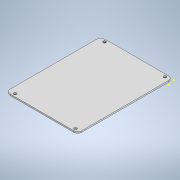
# Autodesk Inventor part: Base
Saved by Autodesk Inventor 2022 (Build 260153000, 153)
## iProperties
Created: 2021-07-02
Part Number: Base
Material: Generic
Document SubType Name: Modeling
Designer: anton
Density: 1 g/cm^3
Appearance: Default
Author: anton
Autodesk Inventor part; units mm, degrees
ref_plane "YZ Plane" through (0, 0, 0) normal (1, 0, 0) x (0, 1, 0)
ref_plane "XZ Plane" through (0, 0, 0) normal (0, 1, 0) x (-1, 0, 0)
ref_plane "XY Plane" through (0, 0, 0) normal (0, 0, 1) x (1, 0, 0)
sketch "Sketch9" plane through (0, 0, 0) normal (0, 1, 0) x (-1, 0, 0)
  line L0 (21.5945, 0.4535) -> (21.5945, 2.4535)
  line L1 (17.5945, 2.4535) -> (21.5945, 2.4535)
  line L2 (17.5945, 2.4535) -> (17.5945, 10.4535)
  line L3 (17.5945, 10.4535) -> (4.5945, 10.4535)
  line L4 (4.5945, 183.6535) -> (4.5945, 10.4535)
  line L5 (4.5945, 183.6535) -> (17.5945, 183.6535)
  line L6 (17.5945, 183.6535) -> (17.5945, 191.6535)
  line L7 (128.8958, 191.6535) -> (17.5945, 191.6535)
  line L8 (128.8958, 191.6535) -> (128.8958, 183.6535)
  line L9 (128.8958, 183.6535) -> (145.8958, 183.6535)
  line L10 (145.8958, 183.6535) -> (145.8958, 77.6035)
  line L11 (145.8958, 77.6035) -> (148.4777, 77.6035)
  line L12 (148.4777, 77.6035) -> (148.4777, 185.6535)
  ellipse E0 centre (138.5419, 185.6535) end of major axis (148.4777, 185.6535) minor radius 8 (148.4777, 185.6535) -> (138.5419, 193.6535) ccw
  line L13 (138.5419, 193.6535) -> (11.132, 193.6535)
  ellipse E1 centre (11.132, 185.6535) end of major axis (2.4153, 185.6535) minor radius 8 (11.132, 193.6535) -> (2.4153, 185.6535) ccw
  line L14 (2.4153, 8.4535) -> (2.4153, 185.6535)
  ellipse E2 centre (11.132, 8.4535) end of major axis (2.4153, 8.4535) minor radius 8 (2.4153, 8.4535) -> (11.132, 0.4535) ccw
  line L15 (11.132, 0.4535) -> (21.5945, 0.4535)
  circle A0 centre (135.4777, 188.1535) radius 2.9
  circle A1 centre (12.4153, 5.9535) radius 2.9
  circle A2 centre (12.4153, 188.1535) radius 2.9
  line L16 (46.5945, 2.4535) -> (46.5945, 0.4535)
  line L17 (46.5945, 0.4535) -> (138.5419, 0.4535)
  ellipse E3 centre (138.5419, 8.4535) end of major axis (128.606, 8.4535) minor radius 8 (138.5419, 0.4535) -> (148.4777, 8.4535) ccw
  line L18 (148.4777, 8.4535) -> (148.4777, 10.4535)
  line L19 (148.4777, 10.4535) -> (128.8958, 10.4535)
  line L20 (128.8958, 10.4535) -> (128.8958, 2.4535)
  line L21 (46.5945, 2.4535) -> (128.8958, 2.4535)
  circle A3 centre (135.4777, 5.9535) radius 2.9
  point P0 (0, 0)
  point P1 (98.6744, 193.6535)
  constraints: 44 end point, 4 centre point, 16 other
extrude "Extrusion8" add sketch "Sketch9" along normal blind 3
sketch "Sketch12" plane through (0, 3, 0) normal (0, 1, 0) x (1, 0, 0)
  line L0 (-17.5945, -183.6535) -> (-17.5945, -191.6535) projected
  line L1 (-17.5945, -191.6535) -> (-128.8958, -191.6535) projected
  line L2 (-128.8958, -191.6535) -> (-128.8958, -183.6535) projected
  line L3 (-128.8958, -183.6535) -> (-145.8958, -183.6535) projected
  line L4 (-145.8958, -183.6535) -> (-145.8958, -77.6035) projected
  line L5 (-145.8958, -77.6035) -> (-148.4777, -77.6035) projected
  line L6 (-148.4777, -77.6035) -> (-148.4777, -185.6535) projected
  ellipse E0 centre (-138.5419, -185.6535) end of major axis (-148.4777, -185.6535) minor radius 8 (-148.4777, -185.6535) -> (-138.5419, -193.6535) ccw projected
  line L7 (-138.5419, -193.6535) -> (-11.132, -193.6535) projected
  ellipse E1 centre (-11.132, -185.6535) end of major axis (-2.4153, -185.6535) minor radius 8 (-11.132, -193.6535) -> (-2.4153, -185.6535) ccw projected
  line L8 (-2.4153, -185.6535) -> (-2.4153, -8.4535) projected
  ellipse E2 centre (-11.132, -8.4535) end of major axis (-2.4153, -8.4535) minor radius 8 (-2.4153, -8.4535) -> (-11.132, -0.4535) ccw projected
  line L9 (-11.132, -0.4535) -> (-21.5945, -0.4535) projected
  line L10 (-21.5945, -0.4535) -> (-21.5945, -2.4535) projected
  line L11 (-21.5945, -2.4535) -> (-17.5945, -2.4535) projected
  line L12 (-17.5945, -2.4535) -> (-17.5945, -10.4535) projected
  line L13 (-17.5945, -10.4535) -> (-4.5945, -10.4535) projected
  line L14 (-4.5945, -10.4535) -> (-4.5945, -183.6535) projected
  line L15 (-4.5945, -183.6535) -> (-17.5945, -183.6535) projected
  circle A0 centre (-135.4777, -188.1535) radius 2.9 projected
  circle A1 centre (-12.4153, -5.9535) radius 2.9 projected
  circle A2 centre (-12.4153, -188.1535) radius 2.9 projected
  line L16 (-46.5945, -0.4535) -> (-138.5419, -0.4535) projected
  ellipse E3 centre (-138.5419, -8.4535) end of major axis (-128.606, -8.4535) minor radius 8 (-138.5419, -0.4535) -> (-148.4777, -8.4535) ccw projected
  line L17 (-148.4777, -8.4535) -> (-148.4777, -10.4535) projected
  line L18 (-148.4777, -10.4535) -> (-128.8958, -10.4535) projected
  line L19 (-128.8958, -10.4535) -> (-128.8958, -2.4535) projected
  line L20 (-128.8958, -2.4535) -> (-46.5945, -2.4535) projected
  line L21 (-46.5945, -2.4535) -> (-46.5945, -0.4535) projected
  circle A3 centre (-135.4777, -5.9535) radius 2.9 projected
  line L22 (-148.4777, -77.6035) -> (-148.4777, -185.6535) projected
  line L23 (-148.4777, -77.6035) -> (-148.4777, -10.4535)
  line L24 (-46.5945, -0.4535) -> (-138.5419, -0.4535) projected
  line L25 (-11.132, -0.4535) -> (-21.5945, -0.4535) projected
  line L26 (-46.5945, -0.4535) -> (-21.5945, -0.4535)
  point P0 (0, 0)
  constraints: 4 end point, 2 collinear, 4 other
extrude "Extrusion9" add sketch "Sketch12" along normal blind 3
sketch "Sketch14" plane through (0, 3, 0) normal (0, -1, 0) x (1, 0, 0)
  line L0 (-148.4777, 8.4535) -> (-148.4777, 10.4535) projected
  line L1 (-148.4777, 10.4535) -> (-76.8917, 10.4535)
  line L2 (-76.8917, 10.4535) -> (-76.8917, 77.6035)
  line L3 (-76.8917, 77.6035) -> (-148.4777, 77.6035)
  line L4 (-148.4777, 77.6035) -> (-148.4777, 10.4535)
  circle A0 centre (-136.5827, 69.7935) radius 4
  circle A1 centre (-139.8757, 18.2635) radius 4
  circle A2 centre (-85.5757, 18.2635) radius 4
  circle A3 centre (-86.4447, 69.1635) radius 4
  point P0 (0, 0)
  dimension "d72" = 71.586
  dimension "d73" = 67.15
  dimension "d74" = 8
  dimension "d75" = 8
  dimension "d76" = 8
  dimension "d77" = 8
  dimension "d78" = 7.81
  dimension "d79" = 11.895
  dimension "d80" = 8.44
  dimension "d81" = 9.553
  dimension "d82" = 7.81
  dimension "d83" = 8.684
  dimension "d84" = 7.81
  dimension "d85" = 8.602
  constraints: 8 end point, 4 centre point, 2 parallel, 1 horizontal, 1 perpendicular
  measures "d72" distance between parallel lines of L4 L2
  measures "d73" distance between parallel lines of L1 L3
  measures "d74" diameter of A3
  measures "d75" diameter of A2
  measures "d76" diameter of A1
  measures "d77" diameter of A0
  measures "d78" distance from line of A0.centre L3
  measures "d79" distance from line of L4 A0.centre
  measures "d80" distance from line of L3 A3.centre
  measures "d81" distance from line of L2 A3.centre
  measures "d82" distance from line of L1 A2.centre
  measures "d83" distance from line of L2 A2.centre
  measures "d84" distance from line of L1 A1.centre
  measures "d85" distance from line of L4 A1.centre
extrude "Extrusion10" add sketch "Sketch14" along normal blind 3 contours A0 | A1 | A2 | A3
sketch "Sketch15" plane through (0, 3, 0) normal (0, -1, 0) x (1, 0, 0)
  line L0 (-148.4777, 10.4535) -> (-128.8958, 10.4535) projected
  line L1 (-145.8958, 77.6035) -> (-148.4777, 77.6035) projected
  line L2 (-145.9777, 10.4535) -> (-148.4777, 10.4535)
  line L3 (-148.4777, 10.4535) -> (-148.4777, 77.6035)
  line L4 (-148.4777, 77.6035) -> (-145.9777, 77.6035)
  line L5 (-145.9777, 77.6035) -> (-145.9777, 10.4535)
  point P0 (0, 0)
  dimension "d88" = 2.5
  constraints: 8 end point, 2 parallel, 1 horizontal, 1 perpendicular, 1 point on line
  measures "d88" distance between parallel lines of L3 L5
extrude "Extrusion11" add sketch "Sketch15" along normal blind 3
sketch "Sketch16" plane through (0, 0, 0) normal (0, -1, 0) x (1, 0, 0)
  line L0 (-148.4777, 8.4535) -> (-148.4777, 185.6535) projected
  line L1 (-148.4777, 10.4784) -> (-147.4777, 10.4784)
  line L2 (-147.4777, 10.4784) -> (-147.4777, 77.6035)
  line L3 (-147.4777, 77.6035) -> (-148.4777, 77.6035)
  line L4 (-148.4777, 77.6035) -> (-148.4777, 10.4784)
  point P0 (0, 0)
  point P1 (-145.8958, 77.6035)
  dimension "d91" = 1
  constraints: 8 end point, 2 parallel, 1 horizontal, 1 perpendicular, 1 point on line
  measures "d91" distance between parallel lines of L0 L2
extrude "Extrusion12" add sketch "Sketch16" along normal blind 1.5
sketch "Sketch17" plane through (0, 0, 0) normal (0, -1, 0) x (1, 0, 0)
  line L0 (-145.9777, 10.4535) -> (-145.9777, 77.6035) projected
  line L1 (-148.4777, 77.6035) -> (-148.4777, 10.4784) projected
  line L2 (-145.9777, 10.4535) -> (-148.4777, 10.4535)
  line L3 (-148.4777, 10.4535) -> (-148.4777, 19.4535)
  line L4 (-148.4777, 19.4535) -> (-145.9777, 19.4535)
  line L5 (-145.9777, 19.4535) -> (-145.9777, 10.4535)
  line L6 (-145.9777, 77.6035) -> (-148.4777, 77.6035)
  line L7 (-148.4777, 77.6035) -> (-148.4777, 71.9535)
  line L8 (-148.4777, 71.9535) -> (-145.9777, 71.9535)
  line L9 (-145.9777, 71.9535) -> (-145.9777, 77.6035)
  point P0 (0, 0)
  dimension "d94" = 5.65
  dimension "d95" = 9
  constraints: 16 end point, 4 parallel, 2 horizontal, 2 perpendicular, 2 point on line
  measures "d94" distance between parallel lines of L8 L6
  measures "d95" distance between parallel lines of L2 L4
extrude "Extrusion13" add sketch "Sketch17" along normal blind 11.17 contours L2 L3 L1 L4 L0 | L8 L1 L6 L0
sketch "Sketch18" plane through (-145.9777, 3, 77.6035) normal (1, 0, 0) x (0, 0, -1)
  line L0 (67.15, -14.17) -> (58.15, -14.17) projected
  line L1 (67.15, -3) -> (67.15, -14.17) projected
  line L2 (58.15, -14.17) -> (67.15, -14.17)
  line L3 (67.15, -14.17) -> (67.15, -12.17)
  line L4 (67.15, -12.17) -> (58.15, -12.17)
  line L5 (58.15, -12.17) -> (58.15, -14.17)
  line L6 (5.65, -14.17) -> (0, -14.17) projected
  line L7 (0, -3) -> (0, -14.17) projected
  line L8 (5.65, -14.17) -> (0, -14.17)
  line L9 (0, -14.17) -> (0, -12.17)
  line L10 (0, -12.17) -> (5.65, -12.17)
  line L11 (5.65, -12.17) -> (5.65, -14.17)
  point P0 (77.6035, -3)
  dimension "d98" = 2
  dimension "d99" = 2
  constraints: 16 end point, 4 parallel, 2 horizontal, 2 perpendicular, 2 point on line
  measures "d98" distance between parallel lines of L6 L10
  measures "d99" distance between parallel lines of L0 L4
extrude "Extrusion14" add sketch "Sketch18" along normal blind 2.5
sketch "Sketch19" plane through (-145.9777, 0, 10.4535) normal (0, 0, -1) x (-1, 0, 0)
  point P0 (-145.9777, 0)
  point P1 (-2.5, -11.17)
sketch "Sketch21" plane through (0, 3, 0) normal (0, -1, 0) x (1, 0, 0)
  line L0 (-145.9777, 77.6035) -> (-145.9777, 10.4535) projected
  line L1 (-145.9777, 10.4535) -> (-128.8958, 10.4535) projected
  line L2 (-128.8958, 10.4535) -> (-128.8958, 2.4535) projected
  line L3 (-128.8958, 2.4535) -> (-46.5945, 2.4535) projected
  line L4 (-46.5945, 2.4535) -> (-46.5945, 0.4535) projected
  line L5 (-21.5945, 0.4535) -> (-46.5945, 0.4535) projected
  line L6 (-21.5945, 0.4535) -> (-21.5945, 2.4535) projected
  line L7 (-21.5945, 2.4535) -> (-17.5945, 2.4535) projected
  line L8 (-17.5945, 2.4535) -> (-17.5945, 10.4535) projected
  line L9 (-17.5945, 10.4535) -> (-4.5945, 10.4535) projected
  line L10 (-4.5945, 10.4535) -> (-4.5945, 183.6535) projected
  line L11 (-4.5945, 183.6535) -> (-17.5945, 183.6535) projected
  line L12 (-17.5945, 183.6535) -> (-17.5945, 191.6535) projected
  line L13 (-17.5945, 191.6535) -> (-128.8958, 191.6535) projected
  line L14 (-128.8958, 191.6535) -> (-128.8958, 183.6535) projected
  line L15 (-128.8958, 183.6535) -> (-145.8958, 183.6535) projected
  line L16 (-145.8958, 183.6535) -> (-145.8958, 77.6035) projected
  line L17 (-145.8958, 77.6035) -> (-145.9777, 77.6035) projected
  circle A0 centre (-139.8757, 18.2635) radius 4 projected
  circle A1 centre (-136.5827, 69.7935) radius 4 projected
  circle A2 centre (-85.5757, 18.2635) radius 4 projected
  circle A3 centre (-86.4447, 69.1635) radius 4 projected
  line L18 (-6.5945, 181.6535) -> (-6.5945, 12.4535)
  line L19 (-6.5945, 12.4535) -> (-19.5945, 12.4535)
  line L20 (-19.5945, 12.4535) -> (-19.5945, 4.4535)
  line L21 (-19.5945, 4.4535) -> (-23.5945, 4.4535)
  line L22 (-44.5945, 4.4535) -> (-126.8958, 4.4535)
  line L23 (-126.8958, 4.4535) -> (-126.8958, 12.4535)
  line L24 (-126.8958, 12.4535) -> (-143.9777, 12.4535)
  line L25 (-143.9777, 12.4535) -> (-143.9777, 75.6035)
  line L26 (-143.9777, 75.6035) -> (-143.8958, 75.6035)
  line L27 (-143.8958, 75.6035) -> (-143.8958, 181.6535)
  line L28 (-143.8958, 181.6535) -> (-126.8958, 181.6535)
  line L29 (-126.8958, 181.6535) -> (-126.8958, 189.6535)
  line L30 (-126.8958, 189.6535) -> (-19.5945, 189.6535)
  line L31 (-19.5945, 189.6535) -> (-19.5945, 181.6535)
  line L32 (-19.5945, 181.6535) -> (-6.5945, 181.6535)
  line L33 (-145.9777, 77.6035) -> (-143.4777, 77.6035) projected
  line L34 (-145.9777, 77.6035) -> (-145.9777, 71.9535) projected
  line L35 (-143.8958, 77.6035) -> (-145.9777, 77.6035)
  line L36 (-138.4447, 12.4535) -> (-138.4447, 10.4535)
  line L37 (-145.9777, 10.4535) -> (-128.8958, 10.4535) projected
  line L38 (-23.5945, 4.4535) -> (-44.5945, 4.4535)
  line L39 (-21.5945, 0.4535) -> (-21.5945, 2.4535) projected
  line L40 (-21.5945, 2.4535) -> (-46.5945, 2.4535)
  point P0 (0, 0)
  dimension "d112" = 2
  constraints: 38 end point, 4 point on line, 2 horizontal, 2 perpendicular, 13 other
  measures "d112" distance between parallel lines of L10 L18
extrude "Extrusion16" add sketch "Sketch21" along normal blind 2 contours L16 L15 L14 L13 L12 L11 L10 L9 L8 L7 L40 L3 L2 L1 L36 L24 L23 L22 L38 L21 L20 L19 L18 L32 L31 L30 L29 L28 L27 L33
sketch "Sketch22" plane through (0, 0, 0) normal (0, -1, 0) x (1, 0, 0)
  line L0 (-148.4777, 77.6035) -> (-145.9777, 77.6035) projected
  line L1 (-145.8958, 77.6035) -> (-145.9777, 77.6035) projected
  line L2 (-145.8958, 183.6535) -> (-145.8958, 77.6035) projected
  line L3 (-128.8958, 183.6535) -> (-145.8958, 183.6535) projected
  line L4 (-128.8958, 191.6535) -> (-128.8958, 183.6535) projected
  line L5 (-17.5945, 191.6535) -> (-128.8958, 191.6535) projected
  line L6 (-17.5945, 183.6535) -> (-17.5945, 191.6535) projected
  line L7 (-4.5945, 183.6535) -> (-17.5945, 183.6535) projected
  line L8 (-4.5945, 10.4535) -> (-4.5945, 183.6535) projected
  line L9 (-17.5945, 10.4535) -> (-4.5945, 10.4535) projected
  line L10 (-17.5945, 2.4535) -> (-17.5945, 10.4535) projected
  line L11 (-21.5945, 2.4535) -> (-17.5945, 2.4535) projected
  line L12 (-21.5945, 0.4535) -> (-21.5945, 2.4535) projected
  line L13 (-11.132, 0.4535) -> (-21.5945, 0.4535) projected
  ellipse E0 centre (-11.132, 8.4535) end of major axis (-2.4153, 8.4535) minor radius 8 (-11.132, 0.4535) -> (-2.4153, 8.4535) ccw projected
  line L14 (-2.4153, 185.6535) -> (-2.4153, 8.4535) projected
  ellipse E1 centre (-11.132, 185.6535) end of major axis (-2.4153, 185.6535) minor radius 8 (-2.4153, 185.6535) -> (-11.132, 193.6535) ccw projected
  line L15 (-138.5419, 193.6535) -> (-11.132, 193.6535) projected
  ellipse E2 centre (-138.5419, 185.6535) end of major axis (-148.4777, 185.6535) minor radius 8 (-138.5419, 193.6535) -> (-148.4777, 185.6535) ccw projected
  line L16 (-148.4777, 77.6035) -> (-148.4777, 185.6535) projected
  circle A0 centre (-135.4777, 188.1535) radius 2.9 projected
  circle A1 centre (-12.4153, 5.9535) radius 2.9 projected
  circle A2 centre (-12.4153, 188.1535) radius 2.9 projected
  line L17 (-145.9777, 10.4535) -> (-148.4777, 10.4535) projected
  line L18 (-148.4777, 8.4535) -> (-148.4777, 10.4535) projected
  ellipse E3 centre (-138.5419, 8.4535) end of major axis (-128.606, 8.4535) minor radius 8 (-148.4777, 8.4535) -> (-138.5419, 0.4535) ccw projected
  line L19 (-46.5945, 0.4535) -> (-138.5419, 0.4535) projected
  line L20 (-46.5945, 2.4535) -> (-46.5945, 0.4535) projected
  line L21 (-128.8958, 2.4535) -> (-46.5945, 2.4535) projected
  line L22 (-128.8958, 10.4535) -> (-128.8958, 2.4535) projected
  line L23 (-145.9777, 10.4535) -> (-128.8958, 10.4535) projected
  circle A3 centre (-135.4777, 5.9535) radius 2.9 projected
  point P0 (0, 0)
  constraints: 4 other
extrude "Extrusion17" cut sketch "Sketch22" against normal blind 3
sketch "Sketch23" plane through (0, 3, 0) normal (0, -1, 0) x (1, 0, 0)
  circle A0 centre (-12.4153, 5.9535) radius 2.9 projected
  circle A1 centre (-12.4153, 5.9535) radius 1.5
  circle A2 centre (-135.4777, 5.9535) radius 2.9 projected
  circle A3 centre (-135.4777, 5.9535) radius 1.5
  circle A4 centre (-135.4777, 188.1535) radius 2.9 projected
  circle A5 centre (-135.4777, 188.1535) radius 1.5
  circle A6 centre (-12.4153, 188.1535) radius 2.9 projected
  circle A7 centre (-12.4153, 188.1535) radius 1.5
  circle A8 centre (-135.4777, 188.1535) radius 2.9
  circle A9 centre (-12.4153, 188.1535) radius 2.9
  circle A10 centre (-12.4153, 5.9535) radius 2.9
  circle A11 centre (-135.4777, 5.9535) radius 2.9
  point P0 (0, 0)
  dimension "d117" = 3
  dimension "d118" = 3
  dimension "d119" = 3
  dimension "d120" = 3
  constraints: 8 centre point, 8 coincident, 4 concentric
  measures "d117" diameter of A7
  measures "d118" diameter of A1
  measures "d119" diameter of A3
  measures "d120" diameter of A5
extrude "Extrusion18" add sketch "Sketch23" against normal blind 0.5
sketch "Sketch25" plane through (0, 3, 0) normal (0, -1, 0) x (1, 0, 0)
  circle A0 centre (-45.0945, 5.7535) radius 4
  circle A1 centre (-24.5945, 5.7535) radius 4
  circle A2 centre (-45.0945, 21.2535) radius 4
  circle A3 centre (-24.5945, 21.2535) radius 4
  line L0 (-11.132, 0.4535) -> (-138.5419, 0.4535) projected
  line L1 (-19.5945, 12.4535) -> (-19.5945, 4.4535) projected
  point P0 (0, 0)
  dimension "d123" = 0
  dimension "d124" = 0
  dimension "d125" = 15.5
  dimension "d126" = 0
  dimension "d127" = 20.5
  dimension "d128" = 8
  dimension "d129" = 8
  dimension "d130" = 8
  dimension "d131" = 8
  dimension "d132" = 5.3
  dimension "d133" = 5
  dimension "d134" = 0
  constraints: 4 centre point
  measures "d123" vertical distance of A1.centre A0.centre
  measures "d124" horizontal distance of A2.centre A0.centre
  measures "d125" distance of A1.centre A3.centre
  measures "d126" vertical distance of A3.centre A2.centre
  measures "d127" distance of A1.centre A0.centre
  measures "d128" diameter of A0
  measures "d129" diameter of A2
  measures "d130" diameter of A3
  measures "d131" diameter of A1
  measures "d132" distance from line of L0 A0.centre
  measures "d133" distance from line of L1 A1.centre
  measures "d134" horizontal distance of A1.centre A3.centre
extrude "Extrusion19" add sketch "Sketch25" along normal blind 8
sketch "Sketch26" plane through (-45.0945, -5, 5.7535) normal (0, -1, 0) x (1, 0, 0)
  line L0 (27.5, -3.3) -> (22.7605, -3.3) projected
  line L1 (25.1303, -3.3) -> (-5.6282, -3.3)
  line L2 (-5.6282, -3.3) -> (-5.6282, -9.492)
  line L3 (-5.6282, -9.492) -> (25.1303, -9.492)
  line L4 (25.1303, -9.492) -> (25.1303, -3.3)
  point P0 (45.0945, -5.7535)
  constraints: 8 end point, 2 parallel, 1 horizontal, 1 midpoint, 1 perpendicular
extrude "Extrusion20" cut sketch "Sketch26" against normal blind 8
sketch "Sketch27" plane through (0, -5, 0) normal (0, -1, 0) x (1, 0, 0)
  arc A0 (-22.3339, 2.4535) -> (-26.855, 2.4535) centre (-24.5945, 5.7535) ccw projected
  circle A1 centre (-24.5945, 5.7535) radius 1.5
  circle A2 centre (-24.5945, 21.2535) radius 4 projected
  circle A3 centre (-24.5945, 21.2535) radius 1.5
  circle A4 centre (-45.0945, 21.2535) radius 4 projected
  circle A5 centre (-45.0945, 21.2535) radius 1.5
  arc A6 (-41.3116, 4.4535) -> (-48.8773, 4.4535) centre (-45.0945, 5.7535) ccw projected
  circle A7 centre (-45.0945, 5.7535) radius 1.5
  point P0 (0, 0)
  dimension "d139" = 3
  dimension "d140" = 3
  dimension "d141" = 3
  dimension "d142" = 3
  constraints: 4 centre point, 4 coincident
  measures "d139" diameter of A7
  measures "d140" diameter of A5
  measures "d141" diameter of A3
  measures "d142" diameter of A1
extrude "Extrusion21" cut sketch "Sketch27" against normal blind 6 contours A1 | A3 | A5 | A7
sketch "Sketch32" plane through (0, 3, 0) normal (0, -1, 0) x (1, 0, 0)
  line L0 (-148.4777, 19.4535) -> (-143.4777, 19.4535) projected
  line L1 (-143.4777, 19.4535) -> (-150.8424, 19.4535)
  line L2 (-150.8424, 19.4535) -> (-150.8424, 9.0687)
  line L3 (-150.8424, 9.0687) -> (-143.4777, 9.0687)
  line L4 (-143.4777, 9.0687) -> (-143.4777, 19.4535)
  line L5 (-143.4777, 71.9535) -> (-143.4777, 77.6035) projected
  line L6 (-148.4777, 8.4535) -> (-148.4777, 185.6535) projected
  line L7 (-143.4777, 71.9535) -> (-148.4777, 71.9535)
  line L8 (-148.4777, 71.9535) -> (-148.4777, 77.6185)
  line L9 (-148.4777, 77.6185) -> (-143.4777, 77.6185)
  line L10 (-143.4777, 77.6185) -> (-143.4777, 71.9535)
  point P0 (0, 0)
  point P1 (-148.4777, 9.0687)
  constraints: 16 end point, 4 parallel, 2 horizontal, 2 perpendicular, 1 point on line
extrude "Extrusion24" cut sketch "Sketch32" along normal blind 100 contours L0 L4 L3 L6 | L7 L6 L9 L10 L5
sketch "Sketch33" plane through (0, 0, 0) normal (0, -1, 0) x (1, 0, 0)
  arc A0 (-143.4777, 16.5241) -> (-143.6946, 19.4535) centre (-139.8757, 18.2635) ccw projected
  circle A1 centre (-139.8757, 18.2635) radius 4
  point P0 (0, 0)
  point P1 (-143.6946, 19.4535)
  constraints: 1 centre point, 1 coincident
extrude "Extrusion25" add sketch "Sketch33" against normal up to surface (3 mm away)
sketch "Sketch34" plane through (0, 3, 0) normal (0, -1, 0) x (1, 0, 0)
  point P0 (0, 0)
sketch "Sketch35" plane through (-17.5945, 3, 2.4535) normal (0, 0, -1) x (-1, 0, 0)
  line L0 (23.5, -8) -> (31.5, -8) projected
  line L1 (11, 0) -> (3, 0) projected
  line L2 (24.5005, -8) -> (10.0005, -8)
  line L3 (10.0005, -8) -> (10.0005, 0)
  line L4 (10.0005, 0) -> (24.5005, 0)
  line L5 (24.5005, 0) -> (24.5005, -8)
  line L6 (25.2395, -8) -> (25.2395, -2) projected
  line L7 (9.2605, -2) -> (9.2605, -8) projected
  point P0 (-17.5945, -3)
  point P1 (29.7605, -8)
  point P2 (10.7829, 0)
  point P3 (3.2171, 0)
  dimension "d164" = 14.5
  dimension "d166" = 0.74
  constraints: 8 end point, 2 parallel, 2 point on line, 1 horizontal, 1 perpendicular
  measures "d164" distance between parallel lines of L3 L5
  measures "d166" distance between parallel lines of L7 L3
extrude "Extrusion26" cut sketch "Sketch35" against normal blind 100
sketch "Sketch36" plane through (-139.8757, 0, 18.2635) normal (0, -1, 0) x (1, 0, 0)
  circle A0 centre (54.3, 0) radius 4 projected
  circle A1 centre (54.3, 0) radius 1.5
  circle A2 centre (53.431, 50.9) radius 4 projected
  circle A3 centre (53.431, 50.9) radius 1.5
  circle A4 centre (3.293, 51.53) radius 4 projected
  circle A5 centre (3.293, 51.53) radius 1.5
  circle A6 centre (0, 0) radius 1.5
  point P0 (139.8757, -18.2635)
  dimension "d170" = 3
  dimension "d171" = 3
  dimension "d172" = 3
  dimension "d173" = 3
  constraints: 4 centre point, 4 coincident
  measures "d170" diameter of A6
  measures "d171" diameter of A5
  measures "d172" diameter of A3
  measures "d173" diameter of A1
extrude "Extrusion27" cut sketch "Sketch36" against normal blind 5 contours A1 | A3 | A5 | A6
sketch "Sketch37" plane through (0, 3, 0) normal (0, -1, 0) x (1, 0, 0)
  line L0 (-123.8958, 158.7935) -> (-70.8958, 158.7935)
  line L1 (-70.8958, 158.7935) -> (-70.8958, 83.7935)
  line L2 (-70.8958, 83.7935) -> (-123.8958, 83.7935)
  line L3 (-123.8958, 83.7935) -> (-123.8958, 158.7935)
  circle A0 centre (-116.2958, 85.7935) radius 4
  circle A1 centre (-88.1958, 85.7935) radius 4
  circle A2 centre (-121.7958, 145.0935) radius 4
  circle A3 centre (-72.9958, 144.0935) radius 4
  circle A4 centre (-136.5827, 69.7935) radius 4 projected
  line L4 (-143.8958, 77.6185) -> (-143.8958, 181.6535) projected
  point P0 (0, 0)
  dimension "d176" = 8
  dimension "d177" = 8
  dimension "d178" = 8
  dimension "d179" = 8
  dimension "d180" = 75
  dimension "d181" = 53
  dimension "d182" = 17.3
  dimension "d183" = 2
  dimension "d184" = 2
  dimension "d185" = 7.6
  dimension "d186" = 2.1
  dimension "d187" = 2.1
  dimension "d188" = 14.7
  dimension "d189" = 13.7
  dimension "d190" = 10
  dimension "d191" = 20
  constraints: 8 end point, 4 centre point, 2 parallel, 1 horizontal, 1 perpendicular
  measures "d176" diameter of A2
  measures "d177" diameter of A3
  measures "d178" diameter of A1
  measures "d179" diameter of A0
  measures "d180" distance of L0.end L1.end
  measures "d181" distance of L1.end L2.end
  measures "d182" distance from line of L1 A1.centre
  measures "d183" distance from line of L2 A1.centre
  measures "d184" distance from line of L2 A0.centre
  measures "d185" distance from line of L3 A0.centre
  measures "d186" distance from line of L3 A2.centre
  measures "d187" distance from line of L1 A3.centre
  measures "d188" distance from line of L0 A3.centre
  measures "d189" distance from line of L0 A2.centre
  measures "d190" distance edge to line of A4 L2
  measures "d191" distance between parallel lines of L4 L3
extrude "Extrusion28" add sketch "Sketch37" along normal blind 3 contours A2 L3 | L3 A2 | A3 L1 | L1 A3 | A0 L2 | L2 A0 | A1 L2 | L2 A1
sketch "Sketch38" plane through (-72.9958, 0, 144.0935) normal (0, -1, 0) x (1, 0, 0)
  circle A0 centre (-15.2, -58.3) radius 4 projected
  circle A1 centre (-15.2, -58.3) radius 1.5
  circle A2 centre (-43.3, -58.3) radius 4 projected
  circle A3 centre (-43.3, -58.3) radius 1.5
  circle A4 centre (-48.8, 1) radius 4 projected
  circle A5 centre (-48.8, 1) radius 1.5
  circle A6 centre (0, 0) radius 4 projected
  circle A7 centre (0, 0) radius 1.5
  point P0 (72.9958, -144.0935)
  dimension "d194" = 3
  dimension "d195" = 3
  dimension "d196" = 3
  dimension "d197" = 3
  constraints: 4 centre point, 4 coincident
  measures "d194" diameter of A7
  measures "d195" diameter of A1
  measures "d196" diameter of A3
  measures "d197" diameter of A5
extrude "Extrusion29" cut sketch "Sketch38" against normal blind 5 contours A1 | A3 | A5 | A7
sketch "Sketch39" plane through (0, 3, 0) normal (0, -1, 0) x (1, 0, 0)
  line L0 (-11.132, 0.4535) -> (-138.5419, 0.4535) projected
  line L1 (-64.5945, 0.4535) -> (-50.5945, 0.4535)
  line L2 (-50.5945, 0.4535) -> (-50.5945, 20.4535)
  line L3 (-50.5945, 20.4535) -> (-64.5945, 20.4535)
  line L4 (-64.5945, 20.4535) -> (-64.5945, 0.4535)
  circle A0 centre (-61.7445, 10.4535) radius 4
  circle A1 centre (-53.4445, 10.4535) radius 4
  circle A2 centre (-45.0945, 5.7535) radius 1.5 projected
  point P0 (0, 0)
  dimension "d200" = 8
  dimension "d201" = 8
  dimension "d202" = 8.3
  dimension "d203" = 10
  dimension "d204" = 10
  dimension "d227" = 2.85
  dimension "d228" = 14
  dimension "d229" = 20
  dimension "d230" = 4
  constraints: 8 end point, 2 centre point, 2 parallel, 1 horizontal, 1 perpendicular, 1 point on line
  measures "d200" diameter of A1
  measures "d201" diameter of A0
  measures "d202" distance of A1.centre A0.centre
  measures "d203" distance from line of L0 A0.centre
  measures "d204" distance from line of L0 A1.centre
  measures "d227" distance from line of A1.centre L2
  measures "d228" distance between parallel lines of L4 L2
  measures "d229" distance between parallel lines of L0 L3
  measures "d230" distance edge to line of A2 L2
extrude "Extrusion30" add sketch "Sketch39" along normal blind 1.9 contours A1 L2 | L2 A1 | A0 L4 | L4 A0
sketch "Sketch40" plane through (0, 3, 0) normal (0, -1, 0) x (1, 0, 0)
  arc A0 (-48.8773, 4.4535) -> (-47.355, 2.4535) centre (-45.0945, 5.7535) ccw projected
  line L0 (-48.8773, 4.4535) -> (-126.8958, 4.4535) projected
  line L1 (-126.8958, 4.4535) -> (-126.8958, 12.4535) projected
  line L2 (-126.8958, 12.4535) -> (-138.4447, 12.4535) projected
  line L3 (-138.4447, 12.4535) -> (-138.4447, 10.4535) projected
  line L4 (-128.8958, 10.4535) -> (-138.4447, 10.4535) projected
  line L5 (-128.8958, 2.4535) -> (-128.8958, 10.4535) projected
  line L6 (-47.355, 2.4535) -> (-128.8958, 2.4535) projected
  line L7 (-47.355, 2.4535) -> (-128.8958, 2.4535) projected
  line L8 (-69.7449, 2.4535) -> (-69.7449, 4.4535)
  point P0 (0, 0)
  constraints: 2 end point, 2 point on line, 1 perpendicular
extrude "Extrusion31" cut sketch "Sketch40" along normal blind 10 contours A0 L6 L8 L0
sketch "Sketch41" plane through (-61.7445, 1.1, 10.4535) normal (0, -1, 0) x (1, 0, 0)
  circle A0 centre (8.3, 0) radius 4 projected
  circle A1 centre (8.3, 0) radius 1.5
  circle A2 centre (0, 0) radius 1.5
  point P0 (61.7445, -10.4535)
  dimension "d209" = 3
  dimension "d211" = 3
  constraints: 2 centre point, 1 coincident
  measures "d209" diameter of A1
  measures "d211" diameter of A2
extrude "Extrusion32" cut sketch "Sketch41" against normal blind 4 contours A1 | A2
sketch "Sketch43" plane through (-145.8958, 1, 183.6535) normal (0, 0, 1) x (1, 0, 0)
  line L0 (-2.5819, 2) -> (-2.5819, 5) projected
  line L1 (-2.5819, 2) -> (2.2766, -3.9507)
  line L2 (0.0001, 2) -> (3.723, -2.5599)
  line L3 (0.0001, 2) -> (-2.5819, 2)
  line L4 (0, 0) -> (2, 0) projected
  line L5 (1.633, 0) -> (-0.949, 0)
  point P0 (145.8958, -1)
  dimension "d216" = 129.23
  dimension "d217" = 50.77
  dimension "d218" = 2.582
  constraints: 8 end point, 3 point on line, 1 collinear
  measures "d216" angle of L3 L2
  measures "d217" angle of L3 L1
  measures "d218" distance of L2.start L0.start
extrude "Extrusion33" cut sketch "Sketch43" against normal up to surface (111.7 mm away)
sketch "Sketch44" plane through (0, 3, 0) normal (0, -1, 0) x (1, 0, 0)
  line L0 (-138.4447, 10.4535) -> (-128.8958, 10.4535) projected
  line L1 (-128.8958, 10.4535) -> (-123.8958, 10.4535)
  line L2 (-123.8958, 10.4535) -> (-123.8958, 1.8906)
  line L3 (-123.8958, 1.8906) -> (-128.8958, 1.8906)
  line L4 (-128.8958, 1.8906) -> (-128.8958, 10.4535)
  line L5 (-128.8958, 183.6535) -> (-145.8957, 183.6535) projected
  line L6 (-128.8958, 183.6535) -> (-123.8958, 183.6535)
  line L7 (-123.8958, 183.6535) -> (-123.8958, 192.2419)
  line L8 (-123.8958, 192.2419) -> (-128.8958, 192.2419)
  line L9 (-128.8958, 192.2419) -> (-128.8958, 183.6535)
  line L10 (-128.8958, 183.6535) -> (-128.8958, 191.6535) projected
  point P0 (0, 0)
  dimension "d221" = 8.5884
  dimension "d222" = 5
  dimension "d223" = 5
  dimension "d224" = 0
  constraints: 16 end point, 4 parallel, 2 horizontal, 2 perpendicular, 1 point on line
  measures "d221" distance of L6.end L7.end
  measures "d222" distance between parallel lines of L9 L7
  measures "d223" distance between parallel lines of L4 L2
  measures "d224" distance between parallel lines of L10 L9
extrude "Extrusion34" cut sketch "Sketch44" along normal blind 10
body "Solid3"
